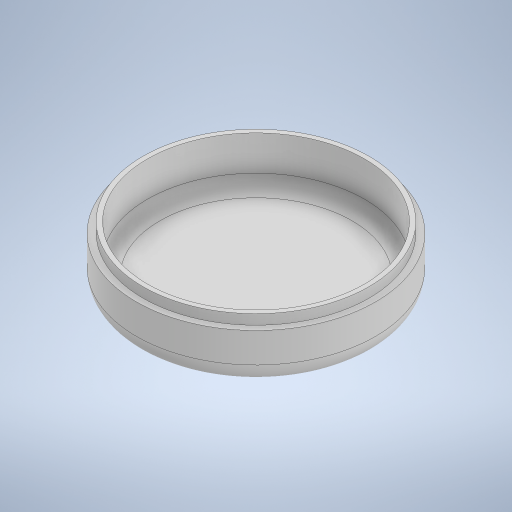
# Autodesk Inventor part: Socle test mesure
Saved by Autodesk Inventor 2024 (Build 280153000, 153)
## iProperties
Created: 2025-01-19
Part Number: Socle test mesure
Material: Générique
Document SubType Name: Modeling
Designer: malam
Density: 1 g/cm^3
Appearance: Par défaut
Author: malam
Autodesk Inventor part; units mm, degrees
ref_plane "YZ Plane" through (0, 0, 0) normal (1, 0, 0) x (0, 1, 0)
ref_plane "XZ Plane" through (0, 0, 0) normal (0, 1, 0) x (-1, 0, 0)
ref_plane "XY Plane" through (0, 0, 0) normal (0, 0, 1) x (1, 0, 0)
sketch "Esquisse1" plane through (0, 0, 0) normal (0, 1, 0) x (-1, 0, 0)
  circle A0 centre (0, 0) radius 45.31
  circle A1 centre (0, 0) radius 47.89
  line L0 (19.5, -32.55) -> (1.5, -32.55)
  line L1 (1.5, -32.55) -> (1.5, 32.55)
  line L2 (1.5, 32.55) -> (19.5, 32.55)
  line L3 (19.5, 32.55) -> (19.5, -32.55)
  line L4 (-1.5, -32.55) -> (-19.5, -32.55)
  line L5 (-19.5, -32.55) -> (-19.5, 32.55)
  line L6 (-19.5, 32.55) -> (-1.5, 32.55)
  line L7 (-1.5, 32.55) -> (-1.5, -32.55)
  line L8 (19.5, -32.55) -> (-19.5, 32.55) construction
  line L9 (19.5, 32.55) -> (-19.5, -32.55) construction
  line L10 (19.5, -32.55) -> (19.5, -43.7402)
  line L11 (19.5, 32.55) -> (19.5, 43.7402)
  point P0 (0, 0)
  point P1 (0, 0)
  dimension "d0" = 90.62
  dimension "d11" = 2.58
  dimension "d16" = 18
  dimension "d17" = 65.1
  dimension "d18" = 18
  dimension "d19" = 3
  constraints: 24 end point, 4 parallel, 2 centre point, 2 horizontal, 2 perpendicular, 2 point on circle, 1 midpoint, 1 point on line, 1 vertical
  measures "d0" diameter of A0
  measures "d11" radial gap between concentric circles of A0 A1
  measures "d16" distance of L1.end L3.start
  measures "d17" distance of L0.end L1.end
  measures "d18" distance of L5.end L7.start
  measures "d19" distance between parallel lines of L7 L1
extrude "Extrusion1" add sketch "Esquisse1" along normal blind 20 contours A0 L11 A1 L10 | A0 L10 A1 L11
sketch "Esquisse4" plane through (0, 0, 0) normal (0, -1, 0) x (1, 0, 0)
  circle A0 centre (0, 0) radius 47.89 projected
  circle A1 centre (0, 0) radius 45.31 projected
extrude "Extrusion4" add sketch "Esquisse4" against normal blind 5 contours A1
fillet "Congé2" radius 8 1 edges at (47.89, 0, 0)
sketch "Esquisse6" plane through (0, 5, 0) normal (0, 1, 0) x (1, 0, 0)
  line L0 (19.5, 32.55) -> (19.5, -32.55) projected
  line L1 (1.5, -32.55) -> (1.5, 32.55) projected
  line L2 (-1.5, 32.55) -> (-1.5, -32.55) projected
  line L3 (-19.5, -32.55) -> (-19.5, 32.55) projected
  line L4 (-19.5, 32.55) -> (-1.5, 32.55) projected
  line L5 (1.5, 32.55) -> (19.5, 32.55) projected
  line L6 (19.5, -32.55) -> (1.5, -32.55) projected
  line L7 (-1.5, -32.55) -> (-19.5, -32.55) projected
  point P0 (0, 0)
sketch "Esquisse7" plane through (0, 20, 0) normal (0, 1, 0) x (1, 0, 0)
  circle A0 centre (0, 0) radius 45.155
  circle A1 centre (0, 0) radius 43.5
  circle A2 centre (0, 0) radius 47.89 projected
  circle A3 centre (0, 0) radius 45.31 projected
  dimension "d35" = 90.31
  dimension "d36" = 87
  constraints: 2 centre point, 2 coincident
  measures "d35" diameter of A0
  measures "d36" diameter of A1
extrude "Extrusion5" add sketch "Esquisse7" against normal up to surface (15 mm away) contours A0 | A3
extrude "Extrusion6" add sketch "Esquisse7" along normal blind 4 contours A0 | A3
fillet "Congé4" radius 5 1 edges at (-43.5, 5, 0)
